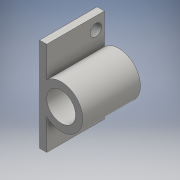
# Autodesk Inventor part: Support endStop v1
Saved by Autodesk Inventor 2016 (Build 200138000, 138)
## iProperties
Created: 2016-07-07
Part Number: Support endStop v1
Material: Generic
Document SubType Name: Modeling
Designer: Thetheos
Density: 1 g/cm^3
Appearance: Default
Author: Thetheos
Autodesk Inventor part; units mm, degrees
ref_plane "YZ Plane" through (0, 0, 0) normal (1, 0, 0) x (0, 1, 0)
ref_plane "XZ Plane" through (0, 0, 0) normal (0, 1, 0) x (-1, 0, 0)
ref_plane "XY Plane" through (0, 0, 0) normal (0, 0, 1) x (1, 0, 0)
sketch "Sketch1" plane through (0, 0, 0) normal (0, 1, 0) x (-1, 0, 0)
  circle A0 centre (0, 0) radius 4
  line L0 (6, 13) -> (4, 13)
  line L1 (6, -13) -> (4, -13)
  arc A1 (4, 4.4721) -> (4, -4.4721) centre (0, 0) ccw
  line L2 (4, 13) -> (4, 4.4721)
  line L3 (4, -4.4721) -> (4, -13)
  line L4 (6, 13) -> (6, -13)
  dimension "d0" = 8
  dimension "d2" = 26
  dimension "d3" = 2
  constraints: 10 end point, 3 point on circle, 3 vertical, 2 centre point, 1 coincident
  measures "d0" diameter of A0
  measures "d2" distance of L1.start L0.start
  measures "d3" distance of L0.start L0.end
extrude "Extrusion1" add sketch "Sketch1" along normal blind 16
sketch "Sketch2" plane through (-6, 0, -13) normal (-1, 0, 0) x (0, 0, 1)
  circle A0 centre (3.35, 13.6) radius 1.6
  circle A1 centre (22.65, 13.6) radius 1.6
  line L0 (8.5279, 16) -> (0, 16) projected
  line L1 (0, 16) -> (26, 16) projected
  point P0 (13, 0)
  dimension "d10" = 3.2
  dimension "d11" = 3.2
  dimension "d14" = 2.4
  dimension "d15" = 2.4
  constraints: 2 centre point
  measures "d10" diameter of A0
  measures "d11" diameter of A1
  measures "d14" distance from line of L0 A0.centre
  measures "d15" distance from line of L1 A1.centre
extrude "Extrusion2" cut sketch "Sketch2" against normal blind 16
body "Solid1"
